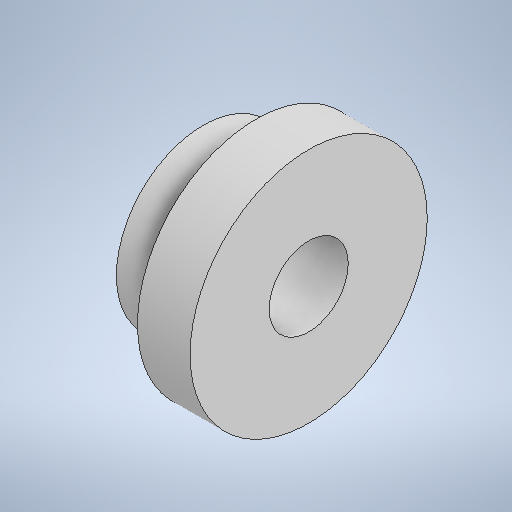
# Autodesk Inventor part: 26-10-210
Saved by Autodesk Inventor 2025.2 (Build 292293000, 293)
## iProperties
Created: 2024-11-14
Part Number: 26-10-210
Material: Generic
Document SubType Name: Modeling
Designer: Zvonko.Gabric
Density: 1 g/cm^3
Appearance: Default
Description: Spring bearing
Author: Zvonko.Gabric
Title: Spring bearing
Subject: Spring bearing
Autodesk Inventor part; units mm, degrees
ref_plane "YZ Plane" through (0, 0, 0) normal (1, 0, 0) x (0, 1, 0)
ref_plane "XZ Plane" through (0, 0, 0) normal (0, 1, 0) x (-1, 0, 0)
ref_plane "XY Plane" through (0, 0, 0) normal (0, 0, 1) x (1, 0, 0)
sketch "Sketch1" plane through (0, 0, 0) normal (0, 1, 0) x (-1, 0, 0)
  line L0 (0, 0) -> (5.9762, 0) construction
  line L1 (0, 0) -> (0, 4.5)
  line L2 (0, 4.5) -> (2, 4.5)
  line L3 (2, 4.5) -> (2, 3.3)
  line L4 (2, 3.3) -> (4, 3.3)
  line L5 (4, 3.3) -> (4, 0)
  line L6 (4, 1.5) -> (0, 1.5)
  dimension "d0" = 4.5
  dimension "d1" = 2
  dimension "d2" = 4
  dimension "d3" = 2
  dimension "d4" = 3.3
  dimension "d5" = 1.5
  constraints: 14 end point, 5 perpendicular, 3 point on line, 1 horizontal, 1 vertical
  measures "d0" distance of L0.start L1.end
  measures "d1" distance of L1.end L2.end
  measures "d2" distance between parallel lines of L1 L5
  measures "d3" distance of L3.end L4.end
  measures "d4" distance between parallel lines of L0 L4
  measures "d5" distance between parallel lines of L0 L6
revolve "Revolution1" add sketch "Sketch1" angle 360 about axis through (0, 0, 0) along (-1, 0, 0)
body "Solid1"
